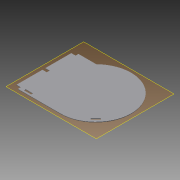
# Autodesk Inventor part: Foam_Left
Saved by Autodesk Inventor 2014 SP1 (Build 180222100, 222)
## iProperties
Created: 2014-02-22
Part Number: Foam_Left
Material: Generic
Document SubType Name: Modeling
Designer: tuleu
Density: 1 g/cm^3
Appearance: Default
Author: tuleu
Autodesk Inventor part; units mm, degrees
ref_plane "YZ Plane" through (0, 0, 0) normal (1, 0, 0) x (0, 1, 0)
ref_plane "XZ Plane" through (0, 0, 0) normal (0, 1, 0) x (-1, 0, 0)
ref_plane "XY Plane" through (0, 0, 0) normal (0, 0, 1) x (1, 0, 0)
ref_plane "Work Plane1" through (0, 0, 0) normal (0, 0, 1) x (1, 0, 0)
sketch "Sketch1" plane through (0, 0, 0) normal (0, 0, 1) x (1, 0, 0)
  arc A0 (185.695, -445.5695) -> (-157.2336, 394.4305) centre (185.695, 44.4305) ccw construction
  arc A1 (185.695, -445.5695) -> (-157.2336, 394.4305) centre (185.695, 44.4305) ccw
  line L0 (-404.305, -445.5695) -> (-404.305, -405.5695) construction
  line L1 (-404.305, -405.5695) -> (-524.305, -405.5695) construction
  line L2 (-524.305, -45.5695) -> (-404.305, -45.5695) construction
  line L3 (-404.305, -45.5695) -> (-404.305, -5.5695) construction
  line L4 (-404.305, -5.5695) -> (-524.305, -5.5695) construction
  line L5 (-524.305, 354.4305) -> (-404.305, 354.4305) construction
  line L6 (-404.305, 354.4305) -> (-404.305, 394.4305) construction
  line L7 (-157.2336, 394.4305) -> (-464.305, 394.4305) construction
  line L8 (-157.2336, 394.4305) -> (-404.305, 394.4305)
  line L9 (-404.305, 354.4305) -> (-464.305, 354.4305)
  line L10 (-464.305, -5.5695) -> (-404.305, -5.5695)
  line L11 (-404.305, -45.5695) -> (-464.305, -45.5695)
  line L12 (-404.305, -45.5695) -> (-404.305, -5.5695)
  line L13 (-404.305, 354.4305) -> (-404.305, 394.4305)
  line L14 (-464.305, 354.4305) -> (-464.305, -5.5695)
  line L15 (-464.305, -45.5695) -> (-464.305, -405.5695)
  line L16 (-464.305, -405.5695) -> (-404.305, -405.5695)
  line L17 (-404.305, -405.5695) -> (-404.305, -445.5695)
  line L18 (-404.305, -445.5695) -> (185.695, -445.5695)
  line L19 (539.2484, -245.4833) -> (475.6088, -309.1229) projected
  arc A2 (468.5377, -309.1229) -> (475.6088, -309.1229) centre (472.0732, -305.5874) ccw projected
  line L20 (468.5377, -309.1229) -> (457.9311, -298.5163) projected
  arc A3 (457.9311, -291.4453) -> (457.9311, -298.5163) centre (461.4666, -294.9808) ccw projected
  line L21 (457.9311, -291.4453) -> (521.5707, -227.8057) projected
  line L22 (528.6418, -227.8057) -> (539.2484, -238.4123) projected
  arc A4 (539.2484, -245.4833) -> (539.2484, -238.4123) centre (535.7128, -241.9478) ccw projected
  arc A5 (528.6418, -227.8057) -> (521.5707, -227.8057) centre (525.1062, -231.3412) ccw projected
  line L23 (-249.305, -420.5695) -> (-339.305, -420.5695) projected
  arc A6 (-249.305, -420.5695) -> (-244.305, -415.5695) centre (-249.305, -415.5695) ccw projected
  line L24 (-244.305, -400.5695) -> (-244.305, -415.5695) projected
  arc A7 (-244.305, -400.5695) -> (-249.305, -395.5695) centre (-249.305, -400.5695) ccw projected
  line L25 (-339.305, -395.5695) -> (-249.305, -395.5695) projected
  arc A8 (-339.305, -395.5695) -> (-344.305, -400.5695) centre (-339.305, -400.5695) ccw projected
  line L26 (-344.305, -415.5695) -> (-344.305, -400.5695) projected
  arc A9 (-344.305, -415.5695) -> (-339.305, -420.5695) centre (-339.305, -415.5695) ccw projected
  point P0 (0, 0)
  constraints: 22 end point, 4 midpoint, 3 collinear, 3 perpendicular, 2 parallel, 2 point on circle, 2 tangent, 1 centre point, 1 coincident
extrude "Extrusion1" add sketch "Sketch1" along normal blind 7
body "Solid1"
